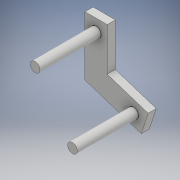
# Autodesk Inventor part: 鸦片
Saved by Autodesk Inventor 2018 (Build 220112000, 112)
## iProperties
Created: 2021-03-02
Part Number: 鸦片
Material: 常规
Document SubType Name: Modeling
Designer: OHHHHHHHHHH
Density: 1 g/cm^3
Appearance: 默认
Author: OHHHHHHHHHH
## iProperties of the stored document 鸦片_3D 打印.ipt
Created: 2021-03-02
Part Number: 鸦片_3D 打印
Material: 常规
Document SubType Name: Modeling
Designer: OHHHHHHHHHH
Density: 1 g/cm^3
Appearance: 默认
Author: OHHHHHHHHHH
Autodesk Inventor part; units mm, degrees
ref_plane "YZ Plane" through (0, 0, 0) normal (1, 0, 0) x (0, 1, 0)
ref_plane "XZ Plane" through (0, 0, 0) normal (0, 1, 0) x (-1, 0, 0)
ref_plane "XY Plane" through (0, 0, 0) normal (0, 0, 1) x (1, 0, 0)
sketch "草图1" plane through (0, 0, 0) normal (0, 1, 0) x (-1, 0, 0)
  circle A0 centre (-2.0908, 11.2121) radius 1.25
  line L0 (-5.7974, 4.2121) -> (1.6092, -1.1691) construction
  circle A1 centre (-11.3094, -1.4762) radius 1.25
  line L1 (0.7195, 14.068) -> (0.7195, -0.5227)
  line L2 (-4.7634, 3.4608) -> (-4.7634, 14.068)
  line L3 (-4.7634, 14.068) -> (0.7195, 14.068)
  line L4 (-13.1571, -5.0315) -> (0.7195, -0.5227)
  line L5 (-4.7634, 3.4608) -> (-14.8514, 0.183)
  line L6 (-14.8514, 0.183) -> (-13.1571, -5.0315)
  dimension "d12" = 2.5
  constraints: 14 end point, 3 symmetric about line, 2 centre point, 2 point on line, 2 vertical, 1 perpendicular, 1 other
  measures "d12" diameter of A0
extrude "拉伸1" add sketch "草图1" along normal blind 2
sketch "草图2" plane through (0, 2, 0) normal (0, 1, 0) x (1, 0, 0)
  circle A0 centre (11.3094, 1.4762) radius 1.25 projected
  circle A1 centre (2.0908, -11.2121) radius 1.25 projected
extrude "拉伸2" add sketch "草图2" against normal blind 2.1
sketch "草图3" plane through (11.3094, -0.1, -1.4762) normal (0, -1, 0) x (1, 0, 0)
  circle A0 centre (-9.2186, 12.6883) radius 1.25 projected
  circle A1 centre (0, 0) radius 1.25 projected
  circle A2 centre (-9.2186, 12.6883) radius 1.2
  circle A3 centre (0, 0) radius 1.2
  point P0 (-11.3094, 1.4762)
  dimension "d13" = 2.4
  dimension "d14" = 2.4
  constraints: 2 centre point
  measures "d13" diameter of A3
  measures "d14" diameter of A2
extrude "拉伸3" add sketch "草图3" along normal blind 15 contours A2 | A3
